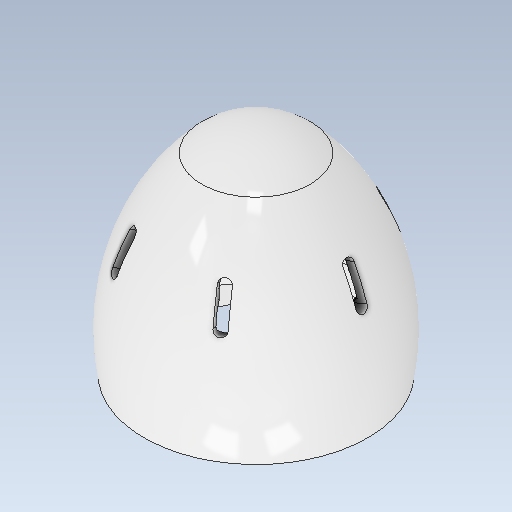
# Autodesk Inventor part: SmartEgg Shell Top
Saved by Autodesk Inventor 2020 (Build 240168000, 168)
## iProperties
Created: 2019-11-26
Part Number: SmartEgg Shell Top
Material: Generic
Document SubType Name: Modeling
Designer: Andrew
Density: 1 g/cm^3
Appearance: White
Author: Andrew
Autodesk Inventor part; units mm, degrees
ref_plane "YZ Plane" through (0, 0, 0) normal (1, 0, 0) x (0, 1, 0)
ref_plane "XZ Plane" through (0, 0, 0) normal (0, 1, 0) x (-1, 0, 0)
ref_plane "XY Plane" through (0, 0, 0) normal (0, 0, 1) x (1, 0, 0)
derived "SmartEgg Shell.ipt"
sketch "Shell Sketch" plane through (0, -9.787, -13.5347) normal (0, 0.8032373, -0.5956591) x (0, 0.5956591, 0.8032373)
  arc A0 (40.7438, -16.765) -> (29.159, 32.4326) centre (-7.0434, -2.0549) ccw
  arc A1 (16.8502, -34.4099) -> (29.3502, -31.0606) centre (16.8502, -9.4099) ccw construction
  line L0 (16.8502, -34.4099) -> (16.8502, -31.0606) construction
  line L1 (16.8502, 9.75) -> (35.7004, 9.75)
  line L2 (16.8502, 26.5) -> (16.8502, -26.5) construction
  line L3 (33.7004, -26.5) -> (34.4025, -27.2121) construction
  arc A2 (29.159, 32.4326) -> (16.8502, 37.7068) centre (16.8502, 20.7068) ccw
  line L4 (16.8502, 37.7068) -> (16.8502, 34.849)
  line L5 (16.8502, 34.849) -> (21.8502, 34.849)
  arc A3 (27.7109, 31.0531) -> (21.8502, 34.849) centre (16.8502, 20.7068) ccw
  arc A4 (37.5734, 15.6465) -> (27.7109, 31.0531) centre (-7.0434, -2.0549) ccw
  arc A5 (33.7004, 22) -> (29.2004, 26.5) centre (29.2004, 22) ccw construction
  line L6 (35.7004, 9.75) -> (35.7004, -11.0606)
  line L7 (35.7004, -11.0606) -> (42.1389, -11.0606)
  line L8 (38.7004, 9.75) -> (38.7004, -10.8106)
  line L9 (38.7004, -10.8106) -> (42.184, -10.8106)
  line L10 (16.8502, -31.0606) -> (29.3502, -31.0606)
  arc A6 (29.3502, -31.0606) -> (40.7438, -16.765) centre (16.8502, -9.4099) ccw
  line L11 (16.8502, -31.0606) -> (16.8502, 9.75)
  line L12 (33.7004, -26.5) -> (33.7004, 22) construction
  line L13 (19.9774, 10.75) -> (16.7013, 10.75) construction
  arc A7 (38.7004, 9.75) -> (37.5734, 15.6465) centre (22.7111, 9.75) ccw
  point P0 (16.7013, 0)
  point P1 (38.7004, 12.4883)
sketch "Thread Sketch" plane through (0, -9.787, -13.5347) normal (0, 0.8032373, -0.5956591) x (0, 0.5956591, 0.8032373)
  line L0 (35.7004, 9.75) -> (35.7004, -11.0606) construction
  line L1 (38.7004, 9.75) -> (38.7004, -10.8106) construction
  line L2 (35.7004, 9.75) -> (38.2004, 7.25)
  line L3 (38.2004, 7.25) -> (38.2004, 5.25)
  line L4 (38.2004, 5.25) -> (35.7004, 2.75)
  line L5 (35.7004, 2.75) -> (35.7004, 9.75)
  line L6 (38.7004, 5.3964) -> (36.2004, 2.8964)
  line L7 (36.2004, 2.8964) -> (36.2004, 0.8964)
  line L8 (36.2004, 0.8964) -> (38.7004, -1.6036)
  line L9 (38.7004, -1.6036) -> (38.7004, 5.3964)
  line L10 (38.2004, 6.25) -> (35.7004, 6.25) construction
  line L11 (36.2004, 1.8964) -> (38.7004, 1.8964) construction
  point P0 (16.7013, 0)
sketch "Thread Mask" plane through (0, -9.787, -13.5347) normal (0, 0.8032373, -0.5956591) x (0, 0.5956591, 0.8032373)
  line L0 (38.7004, 7.25) -> (35.7004, 7.25)
  line L1 (35.7004, 7.25) -> (35.7004, -11.0606)
  line L2 (35.7004, -11.0606) -> (38.7004, -11.0606)
  line L3 (38.7004, -11.0606) -> (38.7004, 7.25)
  line L4 (35.7004, 9.75) -> (35.7004, -11.0606) construction
  line L5 (38.7004, 9.75) -> (38.7004, -10.8106) construction
  point P0 (16.7013, 0)
ref_plane "Vent Plane" through (17.25, 13.4911, 17.8554) normal (-0.3860978, -0.5494704, -0.7409526) x (0.8182033, -0.574929, 0)
sketch "Vent Lookup" plane through (0, -9.787, -13.5347) normal (0, 0.8032373, -0.5956591) x (0, 0.5956591, 0.8032373)
  arc A0 (40.7438, -16.765) -> (29.159, 32.4326) centre (-7.0434, -2.0549) ccw
  line L0 (39.0795, 17.25) -> (16.8502, 7.9458)
  line L1 (16.8502, 26.5) -> (16.8502, -26.5) construction
  line L2 (19.9774, 10.75) -> (16.7013, 10.75) construction
  point P0 (16.7013, 0)
revolve "Revolution1" add sketch "Shell Sketch" angle 360 about axis through (-31.0606, 0.25, 0) along (1, 0, 0) contours L9 L8 A7 A4 A3 L5 L4 A2 A0
coil "Coil1" sketch "Thread Sketch" operation add axis through (-31.0606, 0.25, 0) along (-1, 0, 0) pitch 8.708 turns 3 hand right separate body contours L9 L8 L7 L6
coil "Coil2" sketch "Thread Sketch" operation add axis through (-31.0606, 0.25, 0) along (1, 0, 0) pitch 8.708 turns 3 hand right bodies 2 contours L9 L8 L7 L6
sketch "Top Thread Mask" plane through (0, -9.787, -13.5347) normal (0, 0.8032373, -0.5956591) x (0, 0.5956591, 0.8032373)
  arc A0 (38.7004, 9.75) -> (37.5734, 15.6465) centre (22.7111, 9.75) ccw projected
  arc A1 (37.5734, 15.6465) -> (27.7109, 31.0531) centre (-7.0434, -2.0549) ccw projected
  arc A2 (27.7109, 31.0531) -> (21.8502, 34.849) centre (16.8502, 20.7068) ccw projected
  line L0 (16.8502, 34.849) -> (21.8502, 34.849) projected
  line L1 (16.8502, 34.849) -> (16.8502, -10.8106)
  line L2 (16.8502, -10.8106) -> (38.7004, -10.8106)
  line L3 (38.7004, -10.8106) -> (38.7004, 9.75)
  line L4 (38.7004, -10.8106) -> (42.184, -10.8106) construction
  point P0 (16.7013, 0)
  constraints: 6 end point, 2 vertical, 1 collinear, 1 perpendicular
revolve "Revolution2" cut sketch "Top Thread Mask" angle 360 about axis through (34.849, 0.25, 0) along (-1, 0, 0) keep common part bodies 2
combine bodies "Combine1" operation type add bodies to combine 1 2
sketch "Sketch6" plane through (17.25, 13.4911, 17.8554) normal (-0.3860978, -0.5494704, -0.7409526) x (0.8182033, -0.574929, 0)
  line L0 (-3.3262, 1.7318) -> (3.3262, -1.7318) construction
  line L1 (-3.9034, 0.623) -> (2.7489, -2.8405)
  line L2 (3.9034, -0.623) -> (-2.7489, 2.8405)
  arc A0 (-2.7489, 2.8405) -> (-3.9034, 0.623) centre (-3.3262, 1.7318) ccw
  arc A1 (2.7489, -2.8405) -> (3.9034, -0.623) centre (3.3262, -1.7318) ccw
  line L3 (-31.9152, 16.6165) -> (1.4762, -0.7686) projected
  point P0 (-6.3576, 3.5365)
  point P1 (0, 0)
  point P2 (0, 0)
  point P3 (0, 0)
  point P4 (0, 0)
  dimension "d19" = 2.5
  dimension "d20" = 7.5
  constraints: 8 end point, 4 point on circle, 4 tangent, 2 centre point, 1 coincident, 1 collinear, 1 midpoint, 1 parallel
  measures "d19" distance between parallel lines of L2 L1
  measures "d20" distance of L0.start L0.end
extrude "Extrusion1" add sketch "Sketch6" along normal blind 10 separate body
pattern_circular "Circular Pattern1" count 6 over 360 about axis through (-2.0549, 0.25, 0) along (-1, 0, 0) bodies 3
combine bodies "Combine2" operation type subtract main body 1 bodies to subtract 3
ref_plane "Work Plane2" through (0, -9.787, -13.5347) normal (0, 0.8032373, -0.5956591) x (0, 0.5956591, 0.8032373)
equation "\"d2\" = 2 * Thread_Pitch"
equation "\"d10\" = 2 * Thread_Pitch"
equation "\"Thread_Pitch\" = 4.354"
body "Solid1"
